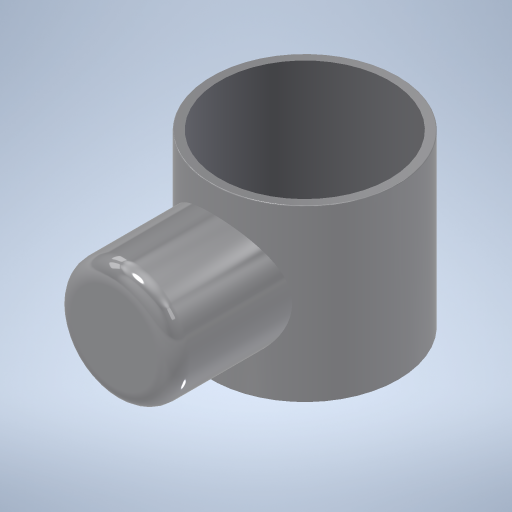
# Autodesk Inventor part: cilindros de dedo gordo
Saved by Autodesk Inventor 2023 (Build 270158000, 158)
## iProperties
Created: 2022-10-12
Part Number: cilindros de dedo gordo
Material: Generic
Document SubType Name: Modeling
Designer: Xiaba
Density: 1 g/cm^3
Appearance: Default
Author: Xiaba
Autodesk Inventor part; units mm, degrees
ref_plane "YZ Plane" through (0, 0, 0) normal (1, 0, 0) x (0, 1, 0)
ref_plane "XY Plane" through (0, 0, 0) normal (0, 0, 1) x (1, 0, 0)
sketch "Sketch1" plane through (0, 0, 0) normal (0, 1, 0) x (-1, 0, 0)
  circle A0 centre (0, 0) radius 1
  circle A1 centre (0, 0) radius 1.1
  dimension "d0" = 2
  dimension "d1" = 2.2
  constraints: 2 centre point, 2 coincident
  measures "d0" diameter of A0
  measures "d1" diameter of A1
extrude "Extrusion1" add sketch "Sketch1" along normal blind 1
sketch "Sketch2" plane through (0, 0, 0) normal (0, 0, 1) x (1, 0, 0)
  line L0 (1.1, 1) -> (-1.1, 1) projected
  line L1 (1.1, 0) -> (-1.1, 0) projected
  line L2 (1.1, 1) -> (-1.1, 1) projected
  line L3 (-1.1, 0) -> (-1.1, 1) projected
  line L4 (1.1, 0) -> (1.1, 1) projected
  line L5 (1.1, 0) -> (-1.1, 0) projected
  circle A0 centre (0, 0.5) radius 0.7
  point P0 (0, 0)
  dimension "d4" = 1.4
  constraints: 1 centre point
  measures "d4" diameter of A0
sketch "Sketch3" plane through (0, 0, 0) normal (0, 1, 0) x (-1, 0, 0)
  circle A0 centre (0, 0) radius 1.1 projected
  circle A1 centre (0, 0) radius 1 projected
ref_plane "Work Plane1" through (0, 0.5, 0) normal (0, 1, 0) x (-1, 0, 0)
sketch "Sketch4" plane through (0, 0.5, 0) normal (0, 1, 0) x (-1, 0, 0)
  circle A0 centre (0, 0) radius 1.1 projected
extrude "Extrusion2" add sketch "Sketch4" along normal mid plane 2
extrude "Extrusion3" add sketch "Sketch2" along normal blind 2.25 contours A0 L1 L0 | L0 A0 | A0 L1
extrude "Extrusion4" cut sketch "Sketch3" along normal through all both and the other way through all contours A1
fillet "Fillet1" radius 0.01 2 edges at (1.1, 1.5, 0) (1, 1.5, 0)
fillet "Fillet2" radius 0.2 1 edges at (-0.7, 0.5, 2.25)
body "Solid1"
